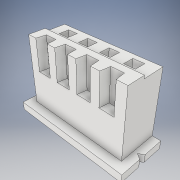
# Autodesk Inventor part: 3S Female JST XH 4 Pin
Saved by Autodesk Inventor 2019.4 (Build 234330000, 330)
## iProperties
Created: 2019-05-09
Part Number: 3S Female JST XH 4 Pin
Material: PBT Plastic
Document SubType Name: Modeling
Designer: JMoll
Density: 1.31 g/cm^3
Appearance: White
Author: JMoll
Autodesk Inventor part; units mm, degrees
ref_plane "YZ Plane" through (0, 0, 0) normal (1, 0, 0) x (0, 1, 0)
ref_plane "XZ Plane" through (0, 0, 0) normal (0, 1, 0) x (-1, 0, 0)
ref_plane "XY Plane" through (0, 0, 0) normal (0, 0, 1) x (1, 0, 0)
sketch "Sketch1" plane through (0, 0, 0) normal (0, 0, 1) x (1, 0, 0)
  line L0 (-5.375, -2) -> (5.375, -2)
  line L1 (5.375, -2) -> (5.375, 2)
  line L2 (5.375, 2) -> (-5.375, 2)
  line L3 (-5.375, 2) -> (-5.375, -2)
  line L4 (-5.375, -2) -> (5.375, 2) construction
  line L5 (5.375, -2) -> (-5.375, 2) construction
  point P0 (0, 0)
  dimension "d0" = 10.75
  dimension "d1" = 4
  constraints: 12 end point, 2 midpoint, 2 parallel, 1 horizontal, 1 perpendicular
  measures "d0" distance of L2.end L1.end
  measures "d1" distance of L2.end L0.start
extrude "Extrusion1" add sketch "Sketch1" along normal blind 7.7
sketch "Sketch2" plane through (0, 0, 0) normal (0, 0, -1) x (-1, 0, 0)
  line L0 (5.375, -2) -> (-5.375, -2) projected
  line L1 (5.375, 2) -> (5.375, -2) projected
  line L2 (-5.375, 2) -> (5.375, 2) projected
  line L3 (-5.375, -2) -> (-5.375, 2) projected
  line L4 (6.25, 2) -> (-6.25, 2)
  line L5 (-6.25, 2) -> (-6.25, -3)
  line L6 (-6.25, -3) -> (6.25, -3)
  line L7 (6.25, -3) -> (6.25, 2)
  point P0 (0, 0)
  dimension "d4" = 0.875
  dimension "d6" = 0.875
  dimension "d7" = 1
  constraints: 8 end point, 2 parallel, 1 horizontal, 1 perpendicular, 1 point on line
  measures "d4" distance between parallel lines of L3 L5
  measures "d6" distance between parallel lines of L7 L1
  measures "d7" distance between parallel lines of L0 L6
extrude "Extrusion2" add sketch "Sketch2" against normal blind 0.9 contours L1 L4 L7 L6 L5 L3 L0
sketch "Sketch3" plane through (0, 0, 7.7) normal (0, 0, 1) x (1, 0, 0)
  line L0 (-5.375, 2) -> (-5.375, -2) projected
  line L1 (5.375, -2) -> (-5.375, -2)
  line L2 (-5.375, -2) -> (-5.375, -0.25)
  line L3 (-5.375, -0.25) -> (5.375, -0.25)
  line L4 (5.375, -0.25) -> (5.375, -2)
  point P0 (0, 0)
  dimension "d10" = 1.75
  constraints: 8 end point, 2 parallel, 1 horizontal, 1 perpendicular, 1 point on line
  measures "d10" distance of L1.end L2.end
extrude "Extrusion3" add sketch "Sketch3" along normal blind 0.3
sketch "Sketch4" plane through (0, 0, 8) normal (0, 0, 1) x (1, 0, 0)
  line L0 (-5.375, -2) -> (5.375, -2) projected
  line L1 (-4.375, -2) -> (-4.25, -1)
  line L2 (-4.25, -1) -> (-3, -1)
  line L3 (-3, -1) -> (-2.875, -2)
  point P0 (0, 0)
  dimension "d13" = 1
  dimension "d14" = 1
  dimension "d15" = 1.5
  dimension "d16" = 1.25
  constraints: 6 end point, 2 point on line, 1 equal length, 1 horizontal
  measures "d13" distance of L0.start L1.start
  measures "d14" distance between parallel lines of L0 L2
  measures "d15" distance of L3.end L1.start
  measures "d16" distance of L1.end L2.end
extrude "Extrusion4" cut sketch "Sketch4" against normal blind 3.25
pattern_linear "Rectangular Pattern1" count 4 spacing 2.4167 along (1, 0, 0) of "Extrusion4"
sketch "Sketch5" plane through (0, 0, 7.7) normal (0, 0, 1) x (1, 0, 0)
  line L0 (-5.375, 2) -> (-5.375, -0.25) projected
  line L1 (-3.075, 0.325) -> (-4.175, 0.325)
  line L2 (-4.175, 0.325) -> (-4.175, 1.425)
  line L3 (-4.175, 1.425) -> (-3.075, 1.425)
  line L4 (-3.075, 1.425) -> (-3.075, 0.325)
  line L5 (-3.075, 0.325) -> (-4.175, 1.425) construction
  line L6 (-4.175, 0.325) -> (-3.075, 1.425) construction
  line L7 (-4.25, -1) -> (-3, -1) projected
  point P0 (0, 0)
  point P1 (-3.625, 0.875)
  point P2 (-3.625, 0.875)
  point P3 (-5.375, 0.875)
  point P4 (-3.625, -1)
  point P5 (-3.625, 0.875)
  dimension "d23" = 1.1
  constraints: 12 end point, 6 midpoint, 2 parallel, 2 perpendicular, 1 horizontal, 1 horizontal alignment, 1 vertical alignment
  measures "d23" distance of L1.end L2.end
extrude "Extrusion5" cut sketch "Sketch5" against normal through all
pattern_linear "Rectangular Pattern2" count 4 spacing 2.4167 along (1, 0, 0) of "Extrusion5"
sketch "Sketch6" plane through (0, 0, 0) normal (0, 0, -1) x (-1, 0, 0)
  line L0 (-2.525, -1.175) -> (-2.525, 1.425)
  line L1 (-2.525, 1.425) -> (-4.725, 1.425)
  line L2 (-4.725, 1.425) -> (-4.725, -1.175)
  line L3 (-4.185, -1.175) -> (-4.185, -1.675)
  line L4 (-4.185, -1.675) -> (-3.065, -1.675)
  line L5 (-3.065, -1.675) -> (-3.065, -1.175)
  line L6 (-4.725, -1.175) -> (-4.185, -1.175)
  line L7 (-3.065, -1.175) -> (-2.525, -1.175)
  line L8 (-4.375, -2) -> (-2.875, -2) projected
  line L9 (-4.25, -1) -> (-4.375, -2) projected
  line L10 (-3, -1) -> (-4.25, -1) projected
  line L11 (-2.875, -2) -> (-3, -1) projected
  line L12 (-1.9583, -2) -> (-0.4583, -2) projected
  line L13 (-1.8333, -1) -> (-1.9583, -2) projected
  line L14 (-0.5833, -1) -> (-1.8333, -1) projected
  line L15 (-0.4583, -2) -> (-0.5833, -1) projected
  point P0 (-3.625, 1.425)
  point P1 (-3.625, -1.675)
  point P2 (-3.625, -1)
  point P3 (-1.2083, -1)
  point P4 (-4.175, 1.425)
  dimension "d31" = 2.2
  dimension "d34" = 1.12
  dimension "d37" = 0.5
  dimension "d38" = 2.6
  dimension "d56" = 2.4167
  constraints: 16 end point, 4 midpoint, 4 parallel, 2 equal length, 2 horizontal, 2 perpendicular, 1 point on line, 1 vertical, 1 vertical alignment
  measures "d31" distance between parallel lines of L2 L0
  measures "d34" distance between parallel lines of L3 L5
  measures "d37" distance between parallel lines of L7 L4
  measures "d38" distance between parallel lines of L1 L7
  measures "d56" distance of point (-3.625, -1) point (-1.208, -1)
sketch "Sketch7" plane through (-5.375, 2, 7.7) normal (0, 1, 0) x (1, 0, 0)
  line L0 (-0.875, 7.7) -> (11.625, 7.7) projected
  line L1 (10.75, 0) -> (0, 0) projected
  line L2 (10.75, 6.8) -> (10.75, 0) projected
  line L3 (8.335, 6.8) -> (9.185, 6.8)
  line L4 (8.335, 3.75) -> (9.985, 3.75)
  line L5 (9.985, 3.75) -> (9.5174, 1.55)
  line L6 (9.5174, 1.55) -> (8.335, 1.55)
  line L7 (8.335, 6.8) -> (8.335, 1.55)
  line L8 (9.185, 6.8) -> (9.585, 3.75)
  line L9 (5.375, 7.7) -> (5.375, 0)
  line L10 (9.185, 6.8) -> (9.067, 7.7)
  line L11 (5.375, 7.7) -> (9.067, 7.7)
  line L12 (8.335, 6.8) -> (5.375, 6.8)
  point P0 (5.375, 7.7)
  dimension "d41" = 0.85
  dimension "d45" = 1.25
  dimension "d46" = 6.15
  dimension "d48" = 2.2
  dimension "d49" = 12
  dimension "d50" = 0.4
  dimension "d52" = 5.92
  dimension "d53" = 0.9
  constraints: 20 end point, 5 point on line, 3 horizontal, 2 midpoint, 2 perpendicular, 1 collinear
  measures "d41" distance of L3.start L3.end
  measures "d45" distance of L4.start L8.end
  measures "d46" distance between parallel lines of L6 L0
  measures "d48" distance between parallel lines of L4 L6
  measures "d49" angle of L2 L5
  measures "d50" distance of L4.end L8.end
  measures "d52" diameter of L7 L9
  measures "d53" distance between parallel lines of L0 L3
extrude "Extrusion6" add sketch "Sketch7" along normal blind 0.85
mirror "Mirror1" about plane through (0, 0, 0) normal (1, 0, 0) of "Extrusion6"
extrude "Extrusion7" cut sketch "Sketch6" against normal blind 4.5 contours L7 L11 L10 L9 L6 L2 L1 L0 | L7 L5 L4 L3 L6 L9 L10 L11
pattern_linear "Rectangular Pattern3" count 4 spacing 2.4167 along (-1, 0, 0) of "Extrusion7"
sketch "Sketch8" plane through (0, 0, 0.9) normal (0, 0, 1) x (1, 0, 0)
  line L0 (6.25, -3) -> (6.25, 2) projected
  line L1 (6.25, -0.85) -> (6.25, -0.15)
  line L2 (6.25, -0.85) -> (5.75, -0.5)
  line L3 (5.75, -0.5) -> (6.25, -0.15)
  point P0 (0, 0)
  point P1 (6.25, -0.5)
  point P2 (6.25, -0.5)
  dimension "d63" = 0.7
  dimension "d64" = 0.5
  constraints: 6 end point, 3 midpoint, 2 point on line, 1 horizontal alignment
  measures "d63" distance of L1.start L1.end
  measures "d64" distance from line of L2.end L0
extrude "Extrusion8" cut sketch "Sketch8" against normal through all
equation "\"d29\" = d21"
equation "\"d61\" = d21"
equation "\"d21\" = 2.416667"
body "Solid1"
